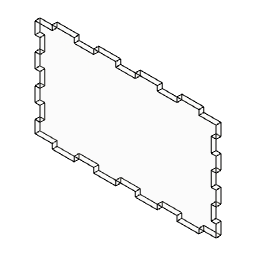
case_5_2mm (Autodesk Fusion 360 design; units mm, degrees)
Autodesk Fusion 360 part; units mm, degrees
sketch "スケッチ1" plane through (0, 0, 0) normal (0, 1, 0) x (1, 0, 0)
  line L0 (0, 0) -> (74, 0)
  line L1 (74, 0) -> (74, -44)
  line L2 (74, -44) -> (0, -44)
  line L3 (0, -44) -> (0, 0)
  dimension "d1" = 74
  dimension "d2" = 44
  constraint horizontal L0
  constraint vertical L1
  constraint horizontal L2
  constraint vertical L3
  constraint coincident L0.start L3.end
  measures "d1" distance of L0.start L0.end
  measures "d2" distance of L0.start L2.end
extrude "押し出し1" add sketch "スケッチ1" along normal blind 2
sketch "スケッチ2" plane through (0, 0, 0) normal (0, -1, 0) x (1, 0, 0)
  line L0 (74, 44) -> (0, 44)
  line L1 (0, 44) -> (0, 0)
  line L2 (0, 0) -> (74, 0)
  line L3 (74, 0) -> (74, 44)
  line L4 (72, 37) -> (74, 37)
  line L5 (74, 37) -> (74, 31)
  line L6 (74, 31) -> (72, 31)
  line L7 (72, 31) -> (72, 37)
  line L8 (74, 25) -> (74, 19)
  line L9 (74, 19) -> (72, 19)
  line L10 (72, 19) -> (72, 25)
  line L11 (72, 25) -> (74, 25)
  line L12 (74, 13) -> (74, 7)
  line L13 (74, 7) -> (72, 7)
  line L14 (72, 7) -> (72, 13)
  line L15 (72, 13) -> (74, 13)
  line L16 (2, 25) -> (2, 19)
  line L17 (2, 31) -> (0, 31)
  line L18 (2, 37) -> (2, 31)
  line L19 (0, 25) -> (2, 25)
  line L20 (2, 13) -> (2, 7)
  line L21 (0, 19) -> (0, 25)
  line L22 (0, 13) -> (2, 13)
  line L23 (2, 7) -> (0, 7)
  line L24 (0, 31) -> (0, 37)
  line L25 (0, 37) -> (2, 37)
  line L26 (0, 7) -> (0, 13)
  line L27 (2, 19) -> (0, 19)
  line L28 (74, 44) -> (72, 44)
  line L29 (72, 44) -> (72, 42)
  line L30 (72, 42) -> (74, 42)
  line L31 (74, 42) -> (74, 44)
  line L32 (0, 44) -> (2, 44)
  line L33 (2, 44) -> (2, 42)
  line L34 (2, 42) -> (0, 42)
  line L35 (0, 42) -> (0, 44)
  line L36 (0, 0) -> (2, 0)
  line L37 (2, 0) -> (2, 2)
  line L38 (2, 2) -> (0, 2)
  line L39 (0, 2) -> (0, 0)
  line L40 (74, 0) -> (72, 0)
  line L41 (72, 0) -> (72, 2)
  line L42 (72, 2) -> (74, 2)
  line L43 (74, 2) -> (74, 0)
  dimension "d7" = 0
  dimension "d8" = -12
  dimension "d9" = 2
  dimension "d10" = 7
  dimension "d11" = 6
  dimension "d12" = 6
  dimension "d13" = 7
  dimension "d16" = -72
  dimension "d17" = 0
  constraint horizontal L4
  constraint vertical L5
  constraint horizontal L6
  constraint vertical L7
  constraint coincident L3 L5.end
  constraint horizontal L28
  constraint vertical L29
  constraint horizontal L30
  constraint vertical L31
  constraint coincident L0.start L3.end
  constraint horizontal L32
  constraint vertical L33
  constraint horizontal L34
  constraint vertical L35
  constraint coincident L0.end L1.start
  constraint horizontal L36
  constraint vertical L37
  constraint horizontal L38
  constraint vertical L39
  constraint coincident L1.end L2.start
  constraint horizontal L40
  constraint vertical L41
  constraint horizontal L42
  constraint vertical L43
  constraint coincident L2.end L3.start
  measures "d9" distance of L4.start L4.end
  measures "d10" distance of L0 L4
  measures "d11" distance of L4.end L5.end
  measures "d12" distance of L6 L11
  measures "d13" distance of L2 L13
extrude "押し出し2" cut sketch "スケッチ2" against normal blind 2 contours L0 L3 L28 L29 L30 L31 | L0 L1 L32 L33 L34 L35 | L3 L4 L5 L6 L7 | L3 L8 L9 L10 L11 | L1 L17 L18 L24 L25 | L3 L12 L13 L14 L15 | L1 L16 L19 L21 L27 | L2 L3 L40 L41 L42 L43 | L1 L20 L22 L23 L26 | L1 L2 L36 L37 L38 L39
sketch "スケッチ3" plane through (0, 0, 0) normal (0, -1, 0) x (1, 0, 0)
  line L0 (74, 31) -> (72, 31)
  line L1 (72, 31) -> (72, 37)
  line L2 (72, 37) -> (74, 37)
  line L3 (74, 37) -> (74, 42)
  line L4 (74, 42) -> (72, 42)
  line L5 (72, 42) -> (72, 44)
  line L6 (72, 44) -> (2, 44)
  line L7 (2, 44) -> (2, 42)
  line L8 (2, 42) -> (0, 42)
  line L9 (0, 42) -> (0, 37)
  line L10 (0, 37) -> (2, 37)
  line L11 (2, 37) -> (2, 31)
  line L12 (2, 31) -> (0, 31)
  line L13 (0, 31) -> (0, 25)
  line L14 (0, 25) -> (2, 25)
  line L15 (2, 25) -> (2, 19)
  line L16 (2, 19) -> (0, 19)
  line L17 (0, 19) -> (0, 13)
  line L18 (0, 13) -> (2, 13)
  line L19 (2, 13) -> (2, 7)
  line L20 (2, 7) -> (0, 7)
  line L21 (0, 7) -> (0, 2)
  line L22 (0, 2) -> (2, 2)
  line L23 (2, 2) -> (2, 0)
  line L24 (2, 0) -> (72, 0)
  line L25 (72, 0) -> (72, 2)
  line L26 (72, 2) -> (74, 2)
  line L27 (74, 2) -> (74, 7)
  line L28 (74, 7) -> (72, 7)
  line L29 (72, 7) -> (72, 13)
  line L30 (72, 13) -> (74, 13)
  line L31 (74, 13) -> (74, 19)
  line L32 (74, 19) -> (72, 19)
  line L33 (72, 19) -> (72, 25)
  line L34 (72, 25) -> (74, 25)
  line L35 (74, 25) -> (74, 31)
  line L36 (0, 44) -> (7, 44)
  line L37 (7, 44) -> (7, 42)
  line L38 (7, 42) -> (0, 42)
  line L39 (0, 42) -> (0, 44)
  line L40 (16, 42) -> (24, 42)
  line L41 (24, 42) -> (24, 44)
  line L42 (24, 44) -> (16, 44)
  line L43 (16, 44) -> (16, 42)
  line L44 (41, 42) -> (41, 44)
  line L45 (33, 42) -> (41, 42)
  line L46 (41, 44) -> (33, 44)
  line L47 (33, 44) -> (33, 42)
  line L48 (58, 42) -> (58, 44)
  line L49 (50, 42) -> (58, 42)
  line L50 (58, 44) -> (50, 44)
  line L51 (50, 44) -> (50, 42)
  line L52 (67, 42) -> (74, 42)
  line L53 (74, 42) -> (74, 44)
  line L54 (74, 44) -> (67, 44)
  line L55 (67, 44) -> (67, 42)
  line L56 (7, 0) -> (0, 0)
  line L57 (41, 2) -> (33, 2)
  line L58 (33, 2) -> (33, 0)
  line L59 (50, 2) -> (50, 0)
  line L60 (24, 2) -> (16, 2)
  line L61 (24, 0) -> (24, 2)
  line L62 (16, 0) -> (24, 0)
  line L63 (7, 2) -> (7, 0)
  line L64 (50, 0) -> (58, 0)
  line L65 (67, 2) -> (67, 0)
  line L66 (0, 0) -> (0, 2)
  line L67 (74, 2) -> (67, 2)
  line L68 (41, 0) -> (41, 2)
  line L69 (58, 2) -> (50, 2)
  line L70 (16, 2) -> (16, 0)
  line L71 (33, 0) -> (41, 0)
  line L72 (67, 0) -> (74, 0)
  line L73 (58, 0) -> (58, 2)
  line L74 (0, 2) -> (7, 2)
  line L75 (74, 0) -> (74, 2)
  line L76 (72, 0) -> (72, 2)
  line L77 (74, 0) -> (72, 0)
  line L78 (2, 2) -> (2, 0)
  line L79 (2, 0) -> (0, 0)
  dimension "d20" = 8
  dimension "d21" = 2
  dimension "d22" = 2
  dimension "d23" = 9
  dimension "d26" = 17
  dimension "d27" = 0
  dimension "d28" = 2
  dimension "d29" = 9
  constraint horizontal L36
  constraint vertical L37
  constraint horizontal L38
  constraint vertical L39
  constraint horizontal L40
  constraint vertical L41
  constraint horizontal L42
  constraint vertical L43
  constraint coincident L6 L41.end
  constraint horizontal L52
  constraint vertical L53
  constraint horizontal L54
  constraint vertical L55
  measures "d20" distance of L40.start L40.end
  measures "d21" distance of L40.start L42.end
  measures "d22" distance of L36.start L8.end
  measures "d23" distance of L37 L43
  measures "d28" distance of L3.end L53.end
  measures "d29" distance of L48 L55
extrude "押し出し3" cut sketch "スケッチ3" against normal blind 2 contours L4 L5 L52 L53 L54 | L5 L6 L52 L54 L55 | L6 L48 L49 L50 L51 | L25 L26 L67 L72 L75 L76 L77 | L6 L44 L45 L46 L47 | L24 L25 L65 L67 L72 L76 | L6 L40 L41 L42 L43 | L24 L59 L64 L69 L73 | L6 L7 L36 L37 L38 | L7 L8 L36 L38 L39 | L24 L57 L58 L68 L71 | L24 L60 L61 L62 L70 | L23 L24 L56 L63 L74 L78 | L22 L23 L56 L66 L74 L78 L79
